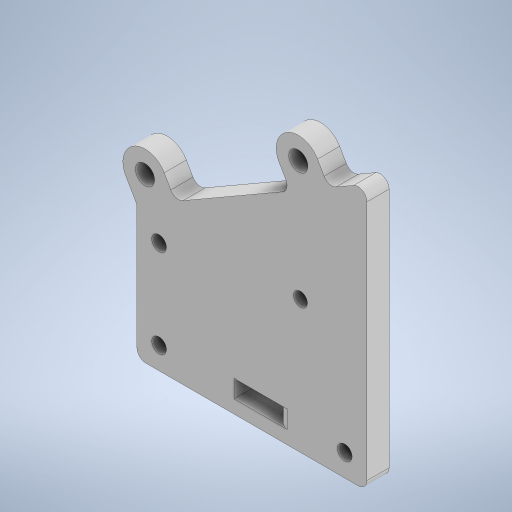
# Autodesk Inventor part: ベースパーツ1
Saved by Autodesk Inventor 2024.3 (Build 283343000, 343)
## iProperties
Created: 2024-10-08
Part Number: ベースパーツ1
Material: 一般
Document SubType Name: Modeling
Designer: hikou
Density: 1 g/cm^3
Appearance: 既定
Author: hikou
Autodesk Inventor part; units mm, degrees
ref_plane "YZ Plane" through (0, 0, 0) normal (1, 0, 0) x (0, 1, 0)
ref_plane "XZ Plane" through (0, 0, 0) normal (0, 1, 0) x (-1, 0, 0)
ref_plane "XY Plane" through (0, 0, 0) normal (0, 0, 1) x (1, 0, 0)
sketch "スケッチ1" plane through (0, 0, 0) normal (0, 0, 1) x (1, 0, 0)
  line L0 (-25.9808, -15) -> (25.9808, -15)
  line L1 (25.9808, -15) -> (25.9808, 15)
  line L2 (25.9808, 15) -> (-25.9808, 15)
  line L3 (-25.9808, 15) -> (-25.9808, -15)
  line L4 (-25.9808, -15) -> (25.9808, 15) construction
  line L5 (25.9808, -15) -> (-25.9808, 15) construction
  line L6 (-25.9808, 15) -> (25.9808, 45)
  line L7 (25.9808, 45) -> (25.9808, 15)
  line L8 (-25.9808, 15) -> (-30.9808, 23.6603)
  line L9 (-30.9808, 23.6603) -> (-22.3205, 28.6603)
  line L10 (-22.3205, 28.6603) -> (-17.3205, 20)
  line L11 (8.6603, 35) -> (3.6603, 43.6603)
  line L12 (3.6603, 43.6603) -> (12.3205, 48.6603)
  line L13 (12.3205, 48.6603) -> (17.3205, 40)
  point P0 (0, 0)
  dimension "d0" = 60
  dimension "d1" = 30
  dimension "d2" = 30
  dimension "d3" = 30
  dimension "d4" = 10
  dimension "d5" = 10
  dimension "d6" = 10
  dimension "d7" = 30
  constraints: 28 end point, 7 perpendicular, 4 point on line, 2 midpoint, 2 parallel, 1 horizontal
  measures "d0" distance of L2.end L6.end
  measures "d1" distance of L6.end L1.end
  measures "d2" angle of L2 L6
  measures "d3" distance of L0.end L1.end
  measures "d4" distance of L2.end L8.end
  measures "d5" distance of L8.end L9.end
  measures "d6" distance of L11.end L12.end
  measures "d7" distance between parallel lines of L10 L11
extrude "押し出し1" add sketch "スケッチ1" along normal mid plane 5
sketch "スケッチ2" plane through (0, 0, 2.5) normal (0, 0, 1) x (1, 0, 0)
  line L0 (-30.9808, 23.6603) -> (-25.9808, 15) projected
  line L1 (-25.9808, 15) -> (-25.9808, -15) projected
  line L2 (-25.9808, -15) -> (25.9808, -15) projected
  line L3 (25.9808, -15) -> (25.9808, 45) projected
  line L4 (25.9808, 45) -> (17.3205, 40) projected
  line L5 (17.3205, 40) -> (12.3205, 48.6603) projected
  line L6 (12.3205, 48.6603) -> (3.6603, 43.6603) projected
  line L7 (3.6603, 43.6603) -> (8.6603, 35) projected
  line L8 (8.6603, 35) -> (-17.3205, 20) projected
  line L9 (-17.3205, 20) -> (-22.3205, 28.6603) projected
  line L10 (-22.3205, 28.6603) -> (-30.9808, 23.6603) projected
  point P0 (0, 0)
  point P1 (-24.1506, 21.8301)
  point P2 (10.4904, 41.8301)
  dimension "d10" = 5
  dimension "d11" = 5
  dimension "d12" = 5
  dimension "d13" = 5
  measures "d10" distance from line of L8 point (-24.151, 21.83)
  measures "d11" distance from line of L8 point (10.49, 41.83)
  measures "d12" distance from line of L9 point (-24.151, 21.83)
  measures "d13" distance from line of point (10.49, 41.83) L7
hole "穴1" at (-24.1506, 21.8301, 2.5) at (10.4904, 41.8301, 2.5) direction (0, 0, -1) diameter 4.3 end through all
sketch "スケッチ4" plane through (0, 0, 2.5) normal (0, 0, 1) x (1, 0, 0)
  line L0 (-25.9808, -15) -> (25.9808, -15) projected
  line L1 (25.9808, -15) -> (25.9808, 45) projected
  point P0 (0, 0)
  point P1 (10.9808, 15)
  dimension "d30" = 30
  dimension "d31" = 15
  measures "d30" distance from line of L0 point (10.981, 15)
  measures "d31" distance from line of L1 point (10.981, 15)
hole "穴2" at (10.9808, 15, 2.5) direction (0, 0, -1) diameter 3.1 end through all
sketch "スケッチ5" plane through (0, 0, 2.5) normal (0, 0, 1) x (1, 0, 0)
  line L0 (-25.9808, 15) -> (-25.9808, -15) projected
  line L1 (-25.9808, -15) -> (25.9808, -15) projected
  line L2 (25.9808, -15) -> (25.9808, 45) projected
  point P0 (0, 0)
  point P1 (-20.9808, 10)
  point P2 (-20.9808, -10)
  point P3 (20.9808, -10)
  dimension "d39" = 5
  dimension "d40" = 5
  dimension "d41" = 5
  dimension "d42" = 20
  dimension "d43" = 5
  dimension "d44" = 5
  measures "d39" distance from line of L0 point (-20.981, -10)
  measures "d40" distance from line of L1 point (-20.981, -10)
  measures "d41" distance from line of L0 point (-20.981, 10)
  measures "d42" distance of point (-20.981, -10) point (-20.981, 10)
  measures "d43" distance from line of L1 point (20.981, -10)
  measures "d44" distance from line of L2 point (20.981, -10)
hole "穴3" at (-20.9808, 10, 2.5) at (-20.9808, -10, 2.5) at (20.9808, -10, 2.5) direction (0, 0, -1) diameter 3.3 end through all
sketch "スケッチ7" plane through (0, 0, -2.5) normal (0, 0, -1) x (-1, 0, 0)
  line L0 (-25.9808, -15) -> (25.9808, -15) projected
  line L1 (-25.9808, 45) -> (-25.9808, -15) projected
  line L2 (-5.9808, -10) -> (4.0192, -10)
  line L3 (4.0192, -10) -> (4.0192, -12)
  line L4 (4.0192, -12) -> (-5.9808, -12)
  line L5 (-5.9808, -12) -> (-5.9808, -10)
  line L6 (-5.9808, -10) -> (4.0192, -10)
  line L7 (4.0192, -10) -> (4.0192, -8)
  line L8 (4.0192, -8) -> (-5.9808, -8)
  line L9 (-5.9808, -8) -> (-5.9808, -10)
  point P0 (0, 0)
  dimension "d52" = 5
  dimension "d53" = 20
  dimension "d54" = 5
  dimension "d55" = 10
  dimension "d56" = 2
  dimension "d57" = 2
  constraints: 16 end point, 5 equal length, 2 perpendicular
  measures "d52" distance from line of L0 L2.start
  measures "d53" distance from line of L1 L2.start
  measures "d54" distance from line of L0 L2.end
  measures "d55" distance of L2.start L2.end
  measures "d56" distance of L2.end L3.end
  measures "d57" distance of L7.end L2.end
extrude "押し出し3" cut sketch "スケッチ7" against normal blind 10
fillet "フィレット1" radius 2 2 edges at (5.9808, -10, 2.5) (5.9808, -10, -2.5)
fillet "フィレット2" radius 2 7 edges at (17.3205, 40, 0) (25.9808, 45, 0) (-17.3205, 20, 0) (8.6603, 35, 0) (-25.9808, 15, 0) (25.9808, -15, 0) (-25.9808, -15, 0)
sketch "スケッチ8" plane through (0, 0, -2.5) normal (0, 0, -1) x (-1, 0, 0)
  arc A0 (23.9808, -15) -> (25.9808, -13) centre (23.9808, -13) ccw projected
  line L0 (25.9808, -13) -> (25.9808, 14.4641) projected
  arc A1 (26.2487, 15.4641) -> (25.9808, 14.4641) centre (27.9808, 14.4641) ccw projected
  line L1 (26.2487, 15.4641) -> (30.9808, 23.6603) projected
  line L2 (30.9808, 23.6603) -> (22.3205, 28.6603) projected
  line L3 (22.3205, 28.6603) -> (18.3205, 21.7321) projected
  arc A2 (15.5885, 21) -> (18.3205, 21.7321) centre (16.5885, 22.7321) ccw projected
  line L4 (15.5885, 21) -> (-6.9282, 34) projected
  arc A3 (-7.6603, 36.7321) -> (-6.9282, 34) centre (-5.9282, 35.7321) ccw projected
  line L5 (-7.6603, 36.7321) -> (-3.6603, 43.6603) projected
  line L6 (-3.6603, 43.6603) -> (-12.3205, 48.6603) projected
  line L7 (-12.3205, 48.6603) -> (-16.3205, 41.7321) projected
  arc A4 (-19.0526, 41) -> (-16.3205, 41.7321) centre (-18.0526, 42.7321) ccw projected
  line L8 (-19.0526, 41) -> (-22.9808, 43.2679) projected
  arc A5 (-22.9808, 43.2679) -> (-25.9808, 41.5359) centre (-23.9808, 41.5359) ccw projected
  line L9 (-25.9808, 41.5359) -> (-25.9808, -13) projected
  arc A6 (-25.9808, -13) -> (-23.9808, -15) centre (-23.9808, -13) ccw projected
  line L10 (-23.9808, -15) -> (23.9808, -15) projected
  circle A7 centre (24.1506, 21.8301) radius 2.15 projected
  circle A8 centre (-10.4904, 41.8301) radius 2.15 projected
  circle A9 centre (-10.9808, 15) radius 1.55 projected
  circle A10 centre (20.9808, 10) radius 1.65 projected
  circle A11 centre (20.9808, -10) radius 1.65 projected
  circle A12 centre (-20.9808, -10) radius 1.65 projected
  line L11 (-7.9808, -8) -> (4.0192, -8) projected
  line L12 (4.0192, -8) -> (4.0192, -12) projected
  line L13 (4.0192, -12) -> (-7.9808, -12) projected
  line L14 (-7.9808, -8) -> (-7.9808, -12) projected
  circle A13 centre (-10.4904, 41.8301) radius 5
  circle A14 centre (24.1506, 21.8301) radius 5
  point P0 (0, 0)
  point P1 (19.8205, 24.3301)
  point P2 (26.6506, 26.1603)
  point P3 (28.4808, 19.3301)
  point P4 (-14.8205, 44.3301)
  point P5 (-7.9904, 46.1603)
  point P6 (-6.1603, 39.3301)
  constraints: 2 centre point, 2 coincident
extrude "押し出し4" cut sketch "スケッチ8" against normal blind 10 contours A14 L2 L1 | L3 L2 A14 | L7 L6 A13 | L6 L5 A13
equation "\"d5\" = d4"
equation "\"d6\" = d4"
equation "\"d11\" = d10"
equation "\"d12\" = d10"
equation "\"d13\" = d10"
equation "\"d40\" = d39"
equation "\"d41\" = d39"
equation "\"d43\" = d39"
equation "\"d44\" = d39"
equation "\"d54\" = d52"
equation "\"d56\" = d57"
